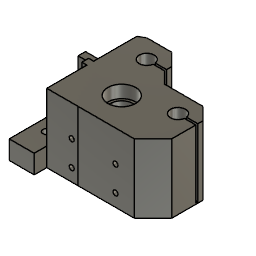
rollos monut left (Autodesk Fusion 360 design; units mm, degrees)
Autodesk Fusion 360 part; units mm, degrees
sketch "Szkic1" plane through (0, 0, 0) normal (0, 0, 1) x (1, 0, 0)
  line L0 (50, 25) -> (25, 25)
  line L1 (-35, -5) -> (-55, -5)
  line L2 (-15, 34.2) -> (0, 34.2)
  line L3 (0, 0) -> (0, -25)
  line L4 (-15.5, -15.5) -> (15.5, 15.5) construction
  line L5 (25, -25) -> (25, 25)
  line L6 (15.5, -15.5) -> (-15.5, 15.5) construction
  line L7 (-30, 25) -> (-30, 50)
  line L8 (-55, -25) -> (-55, -5)
  line L9 (-55, -5) -> (-55, 35)
  circle A0 centre (35, 10) radius 6
  line L10 (50, -5) -> (22, -5)
  line L11 (-25, 25) -> (-30, 25)
  line L12 (35, 9.2) -> (50, 9.2)
  line L13 (-25, -25) -> (-35, -25)
  line L14 (-35, -25) -> (-55, -25)
  line L15 (-40, -12.5) -> (-40, -17.5)
  line L16 (-40, -17.5) -> (-35, -17.5)
  line L17 (-40, -12.5) -> (-35, -12.5)
  line L18 (-15, 35.8) -> (0, 35.8)
  line L19 (-22, 22) -> (22, -22) construction
  line L20 (-25, -25) -> (25, -25)
  line L21 (-30, 50) -> (0, 50)
  line L22 (25, 25) -> (-25, 25)
  line L23 (22, 22) -> (-22, -22) construction
  circle A1 centre (-15, 35) radius 6
  line L24 (-35, -5) -> (-35, -25)
  line L25 (0, 50) -> (0, 25)
  circle A2 centre (-45, -15) radius 3
  line L26 (50, -5) -> (50, 25)
  line L27 (35, 10.8) -> (50, 10.8)
  line L28 (-55, 35) -> (-30, 35)
  line L29 (-25, 25) -> (-25, -25)
  circle A3 centre (0, 0) radius 11.5
  line L30 (-55, -25) -> (-55, -60)
  line L31 (-55, -60) -> (-35, -60)
  line L32 (-35, -60) -> (-35, -25)
  circle A4 centre (-45, -45) radius 3
  line L33 (50, -5) -> (25, -25)
  line L34 (-30, 50) -> (-55, 35)
  line L35 (-25, -25) -> (-25, -60)
  line L36 (-25, -60) -> (-35, -60)
  dimension "d2" = 12
  dimension "d3" = 12
  dimension "d5" = 25
  dimension "d10" = 6
  dimension "d11" = 23
  dimension "d12" = 6
  constraint coincident L3.start L23
  constraint coincident L3.start L19
  constraint perpendicular L11 L29
  constraint perpendicular L7 L11
  constraint perpendicular L7 L21
  constraint midpoint L25.end L22
  constraint perpendicular L22 L25
  constraint perpendicular L3 L20
  constraint vertical L24
  constraint coincident L3.start L6
  constraint coincident L3.start L4
  constraint coincident L6.start L19
  constraint coincident L17.end L24
  constraint perpendicular L17 L24
  constraint coincident L16.end L24
  constraint perpendicular L16 L24
  constraint perpendicular L1 L24
  constraint perpendicular L1 L9
  constraint coincident L28.end L7
  constraint perpendicular L7 L28
  constraint perpendicular L14 L24
  constraint perpendicular L8 L14
  constraint coincident L3.start A3.centre
  constraint perpendicular L14 L30
  constraint perpendicular L30 L31
  constraint perpendicular L14 L32
  constraint perpendicular L13 L35
  constraint perpendicular L32 L36
  measures "d2" diameter of A0
  measures "d3" diameter of A1
  measures "d5" distance of L3.start L3.end
  measures "d10" diameter of A2
  measures "d11" diameter of A3
  measures "d12" diameter of A4
extrude "Wyciągnięcie proste1" add sketch "Szkic1" along normal blind 10 contours L0 L5 A0 L10 L12 L26 L27 | L5 L20 L22 L29 | L5 L10 L33 | L2 L7 L11 L18 L21 L22 A1 L25 | L1 L7 L9 L11 L13 L24 L28 L29 | L13 L32 L35 L36 | L7 L28 L34 makes body 1
extrude "Wyciągnięcie proste2" add sketch "Szkic1" along normal blind 10 contours L15 L16 L17 L24 bodies 1
extrude "Wyciągnięcie proste3" add sketch "Szkic1" against normal blind 10 contours L15 L16 L17 L24 bodies 1
extrude "Wyciągnięcie proste4" add sketch "Szkic1" against normal blind 10 separate body contours L14 L30 L31 L32 makes body 2
extrude "Wyciągnięcie proste5" add sketch "Szkic1" against normal blind 10 contours L1 L8 L14 L15 L16 L17 L24 bodies 1 2
extrude "Wyciągnięcie proste6" add sketch "Szkic1" against normal blind 15 contours L0 L5 A0 L10 L12 L26 L27 | L5 L20 L22 L29 | L5 L10 L33 | L2 L7 L11 L18 L21 L22 A1 L25 | L1 L7 L9 L11 L13 L24 L28 L29 | L13 L32 L35 L36 | L7 L28 L34 bodies 1
sketch "Szkic2" plane through (0, 0, -15) normal (0, 0, -1) x (1, 0, 0)
  circle A0 centre (0, 0) radius 11.5
  line L0 (25, 25) -> (-25, 25)
  line L1 (-25, 25) -> (-25, 60)
  line L2 (-25, 60) -> (-35, 60)
  line L3 (-35, 60) -> (-35, 5)
  line L4 (-35, 5) -> (-55, 5)
  line L5 (-55, 5) -> (-55, -35)
  line L6 (-55, -35) -> (-30, -50)
  line L7 (-30, -50) -> (0, -50)
  line L8 (0, -50) -> (0, -35.8)
  line L9 (0, -35.8) -> (-9.0536, -35.8)
  arc A1 (-9.0536, -34.2) -> (-9.0536, -35.8) centre (-15, -35) ccw
  line L10 (-9.0536, -34.2) -> (0, -34.2)
  line L11 (0, -34.2) -> (0, -25)
  line L12 (0, -25) -> (25, -25)
  line L13 (25, -25) -> (50, -25)
  line L14 (50, -25) -> (50, -10.8)
  line L15 (50, -10.8) -> (40.9464, -10.8)
  arc A2 (40.9464, -9.2) -> (40.9464, -10.8) centre (35, -10) ccw
  line L16 (40.9464, -9.2) -> (50, -9.2)
  line L17 (50, -9.2) -> (50, 5)
  line L18 (50, 5) -> (25, 25)
  circle A3 centre (0, 0) radius 9
  dimension "d25" = 18
  constraint coincident A0.centre A3.centre
  measures "d25" diameter of A3
extrude "Wyciągnięcie proste7" add sketch "Szkic2" against normal blind 15 contours A0 bodies 1
chamfer "Fazowanie1" distance 9.2 angle 45 1 edges at (0, 25, -2.5) on bodies 1
chamfer "Fazowanie2" distance 10 angle 45 1 edges at (50, 25, -2.5) on bodies 1
chamfer "Fazowanie3" distance 10 angle 45 1 edges at (0, 50, -2.5) on bodies 1
chamfer "Fazowanie4" distance 15 angle 45 1 edges at (-25, -25, -2.5) on bodies 1
sketch "Szkic3" plane through (0, 0, 10) normal (0, 0, 1) x (-1, 0, 0)
  line L0 (0, -40) -> (10, -50)
  line L1 (10, -50) -> (30, -50)
  line L2 (30, -50) -> (55, -35)
  line L3 (55, -35) -> (55, 5)
  line L4 (55, 5) -> (35, 5)
  line L5 (35, 5) -> (35, 12.5)
  line L6 (35, 12.5) -> (40, 12.5)
  line L7 (40, 12.5) -> (40, 17.5)
  line L8 (40, 17.5) -> (35, 17.5)
  line L9 (35, 17.5) -> (35, 60)
  line L10 (35, 60) -> (25, 60)
  line L11 (25, 60) -> (25, 40)
  line L12 (25, 40) -> (10, 25)
  line L13 (10, 25) -> (-25, 25)
  line L14 (-25, 25) -> (-50, 5)
  line L15 (-50, 5) -> (-50, -9.2)
  line L16 (-50, -9.2) -> (-40.9464, -9.2)
  arc A0 (-40.9464, -10.8) -> (-40.9464, -9.2) centre (-35, -10) ccw
  line L17 (-40.9464, -10.8) -> (-50, -10.8)
  line L18 (-50, -10.8) -> (-50, -15)
  line L19 (-50, -15) -> (-40, -25)
  line L20 (-40, -25) -> (-25, -25)
  line L21 (-25, -25) -> (-9.2, -25)
  line L22 (-9.2, -25) -> (0, -34.2)
  line L23 (0, -34.2) -> (9.0536, -34.2)
  arc A1 (9.0536, -35.8) -> (9.0536, -34.2) centre (15, -35) ccw
  line L24 (9.0536, -35.8) -> (0, -35.8)
  line L25 (0, -35.8) -> (0, -40)
  circle A2 centre (0, 0) radius 11.5
  line L26 (55, 5) -> (35, 5)
  line L27 (35, 5) -> (35, -5)
  line L28 (35, -5) -> (55, -5)
  line L29 (55, -5) -> (55, 5)
  constraint perpendicular L26 L27
  constraint parallel L26 L28
  constraint parallel L27 L29
  constraint coincident L4.end L5.start
  constraint perpendicular L5 L26
  constraint coincident L3.end L4.start
extrude "Wyciągnięcie proste8" add sketch "Szkic3" along normal blind 25 contours L3 L4 L26 L27 L28 L29 bodies 1
sketch "Szkic4" plane through (0, 5, 0) normal (0, 1, 0) x (-1, 0, 0)
  line L0 (35, 10) -> (55, 10)
  line L1 (55, 10) -> (55, 35)
  line L2 (55, 35) -> (35, 35)
  line L3 (35, 35) -> (35, 10)
  circle A0 centre (45, 25) radius 3
  dimension "d34" = 6
  measures "d34" diameter of A0
extrude "Wyciągnięcie proste9" cut sketch "Szkic4" against normal blind 23 contours A0 bodies 1
chamfer "Fazowanie5" distance 5 angle 45 1 edges at (-45, 5, 10) on bodies 1
sketch "Szkic5" plane through (0, 0, -15) normal (0, 0, -1) x (1, 0, 0)
  circle A0 centre (0, 0) radius 9
  line L0 (-10, -50) -> (0, -40)
  line L1 (0, -40) -> (0, -35.8)
  line L2 (0, -35.8) -> (-9.0536, -35.8)
  arc A1 (-9.0536, -34.2) -> (-9.0536, -35.8) centre (-15, -35) ccw
  line L3 (-9.0536, -34.2) -> (0, -34.2)
  line L4 (0, -34.2) -> (9.2, -25)
  line L5 (9.2, -25) -> (25, -25)
  line L6 (25, -25) -> (40, -25)
  line L7 (40, -25) -> (50, -15)
  line L8 (50, -15) -> (50, -10.8)
  line L9 (50, -10.8) -> (40.9464, -10.8)
  arc A2 (40.9464, -9.2) -> (40.9464, -10.8) centre (35, -10) ccw
  line L10 (40.9464, -9.2) -> (50, -9.2)
  line L11 (50, -9.2) -> (50, 5)
  line L12 (50, 5) -> (25, 25)
  line L13 (25, 25) -> (-10, 25)
  line L14 (-10, 25) -> (-25, 40)
  line L15 (-25, 40) -> (-25, 60)
  line L16 (-25, 60) -> (-35, 60)
  line L17 (-35, 60) -> (-35, 5)
  line L18 (-35, 5) -> (-55, 5)
  line L19 (-55, 5) -> (-55, -35)
  line L20 (-55, -35) -> (-30, -50)
  line L21 (-30, -50) -> (-10, -50)
  line L22 (-9.0536, -34.2) -> (0, -34.2)
  line L23 (0, -34.2) -> (0, -35.8)
  line L24 (0, -35.8) -> (-9.0536, -35.8)
  line L25 (-9.0536, -35.8) -> (-9.0536, -34.2)
  line L26 (40.9464, -9.2) -> (50, -9.2)
  line L27 (50, -9.2) -> (50, -10.8)
  line L28 (50, -10.8) -> (40.9464, -10.8)
  line L29 (40.9464, -10.8) -> (40.9464, -9.2)
  constraint perpendicular L22 L23
  constraint parallel L22 L24
  constraint parallel L23 L25
  constraint coincident L3.end L4.start
  constraint parallel L3 L22
  constraint coincident A1.start L3.start
  constraint perpendicular L26 L27
  constraint parallel L26 L28
  constraint parallel L27 L29
  constraint perpendicular L11 L26
  constraint coincident A2.start L10.start
extrude "Wyciągnięcie proste10" add sketch "Szkic5" against normal blind 1 contours L2 L3 L22 L23 L24 L25 | L9 L10 L26 L27 L28 L29 bodies 1
sketch "Szkic6" plane through (0, -5, 0) normal (0, -1, 0) x (1, 0, 0)
  circle A0 centre (-45, 25) radius 3
  line L0 (-55, 0) -> (-35, 0)
  line L1 (-35, 0) -> (-35, 10)
  line L2 (-35, 10) -> (-35, 35)
  line L3 (-35, 35) -> (-55, 35)
  line L4 (-55, 35) -> (-55, 0)
  line L5 (-46.5, 28) -> (-43.5, 28)
  line L6 (-46.5, 28) -> (-46.5, 27)
  line L7 (-43.5, 28) -> (-43.5, 26.9)
  constraint horizontal L5
  constraint perpendicular L5 L6
  constraint perpendicular L5 L7
extrude "Wyciągnięcie proste11" cut sketch "Szkic6" against normal blind 14.2 contours A0 L5 L7 | A0 L5 L6 bodies 1
sketch "Szkic7" plane through (0, 0, -10) normal (0, 0, -1) x (1, 0, 0)
  circle A0 centre (-45, 15) radius 3
  circle A1 centre (-45, 45) radius 3
  line L0 (-35, 5) -> (-35, 60)
  line L1 (-35, 60) -> (-55, 60)
  line L2 (-55, 60) -> (-55, 5)
  line L3 (-55, 5) -> (-35, 5)
  circle A2 centre (-45, 15) radius 5.5
  circle A3 centre (-45, 45) radius 5.5
  dimension "d42" = 11
  dimension "d43" = 11
  constraint concentric A0 A2
  constraint concentric A1 A3
  measures "d42" diameter of A2
  measures "d43" diameter of A3
extrude "Wyciągnięcie proste12" add sketch "Szkic7" along normal blind 5 contours L0 L1 L2 L3 bodies 1
extrude "Wyciągnięcie proste13" add sketch "Szkic7" along normal blind 0.2 contours A0 | A1 | A2 | A3 bodies 1
sketch "Szkic8" plane through (0, 0, 0) normal (0, 0, 1) x (-1, 0, 0)
  circle A0 centre (0, 0) radius 9
  circle A1 centre (0, 0) radius 11.5
  circle A2 centre (0, 0) radius 11.5
  circle A3 centre (0, 0) radius 11.1
  dimension "d48" = 23
  dimension "d49" = 22.2
  constraint coincident A0.centre A1.centre
  measures "d48" diameter of A2
  measures "d49" diameter of A3
extrude "Wyciągnięcie proste14" add sketch "Szkic8" along normal blind 10 contours A1 A2 bodies 1
extrude "Wyciągnięcie proste15" cut 1 faces at (-45.2225, -5, 10.6917) along direction (0, 1, 0) blind 25 on bodies 1 bodies 1
extrude "Wyciągnięcie proste16" cut 1 faces at (-40, -14.1667, 6.6667) along direction (1, 0, 0) blind 5 on bodies 1 bodies 1
sketch "Szkic9" plane through (0, 0, 0) normal (0, 0, 1) x (-1, 0, 0)
  circle A0 centre (45, 15) radius 3
  circle A1 centre (45, 45) radius 3
  line L0 (35, 60) -> (35, -20)
  line L1 (35, -20) -> (55, -20)
  line L2 (55, -20) -> (55, 60)
  line L3 (55, 60) -> (35, 60)
  circle A2 centre (45, -10) radius 3
  line L4 (35, -12.5) -> (35, -7.1435)
  line L5 (35, -7.1435) -> (39, -7.1435)
  line L6 (39, -7.1435) -> (39, -12.5)
  line L7 (39, -12.5) -> (35, -12.5)
  dimension "d56" = 6
  dimension "d57" = 4
  constraint perpendicular L4 L5
  constraint parallel L4 L6
  constraint parallel L5 L7
  constraint coincident L0 L4.end
  constraint coincident L0 L4.start
  measures "d56" diameter of A2
  measures "d57" distance of L4.start L6.end
extrude "Wyciągnięcie proste17" add sketch "Szkic9" along normal blind 10 contours L0 L4 L5 L6 L7 bodies 1
extrude "Wyciągnięcie proste18" cut sketch "Szkic9" against normal blind 50 contours A2 bodies 1
sketch "Szkic10" plane through (0, 0, 10) normal (0, 0, 1) x (-1, 0, 0)
  line L0 (35, -20) -> (35, -12.5)
  line L1 (35, -12.5) -> (39, -12.5)
  line L2 (39, -12.5) -> (39, -7.1435)
  line L3 (39, -7.1435) -> (35, -7.1435)
  line L4 (35, -7.1435) -> (35, 60)
  line L5 (35, 60) -> (25, 60)
  line L6 (25, 60) -> (25, 40)
  line L7 (25, 40) -> (10, 25)
  line L8 (10, 25) -> (-25, 25)
  line L9 (-25, 25) -> (-50, 5)
  line L10 (-50, 5) -> (-50, -9.2)
  line L11 (-50, -9.2) -> (-40.9464, -9.2)
  arc A0 (-40.9464, -10.8) -> (-40.9464, -9.2) centre (-35, -10) ccw
  line L12 (-40.9464, -10.8) -> (-50, -10.8)
  line L13 (-50, -10.8) -> (-50, -15)
  line L14 (-50, -15) -> (-40, -25)
  line L15 (-40, -25) -> (-25, -25)
  line L16 (-25, -25) -> (-9.2, -25)
  line L17 (-9.2, -25) -> (0, -34.2)
  line L18 (0, -34.2) -> (9.0536, -34.2)
  arc A1 (9.0536, -35.8) -> (9.0536, -34.2) centre (15, -35) ccw
  line L19 (9.0536, -35.8) -> (0, -35.8)
  line L20 (0, -35.8) -> (0, -40)
  line L21 (0, -40) -> (10, -50)
  line L22 (10, -50) -> (30, -50)
  line L23 (30, -50) -> (55, -35)
  line L24 (55, -35) -> (55, -20)
  line L25 (55, -20) -> (35, -20)
  circle A2 centre (0, 0) radius 11.1
  line L26 (55, -20) -> (35, -20)
  line L27 (35, -20) -> (35, -26)
  line L28 (35, -26) -> (55, -26)
  line L29 (55, -26) -> (55, -20)
  dimension "d62" = 6
  constraint perpendicular L26 L27
  constraint parallel L26 L28
  constraint parallel L27 L29
  constraint coincident L0.start L25.end
  constraint parallel L25 L26
  constraint coincident L24.end L25.start
  measures "d62" distance of L24.end L28.end
extrude "Wyciągnięcie proste19" add sketch "Szkic10" along normal blind 20 contours L24 L25 L26 L27 L28 L29 bodies 1
sketch "Szkic11" plane through (0, 26, 0) normal (0, 1, 0) x (-1, 0, 0)
  line L0 (35, 10) -> (55, 10)
  line L1 (55, 10) -> (55, 30)
  line L2 (55, 30) -> (35, 30)
  line L3 (35, 30) -> (35, 10)
  circle A0 centre (45, 20) radius 3
  dimension "d65" = 6
  measures "d65" diameter of A0
extrude "Wyciągnięcie proste20" cut sketch "Szkic11" against normal blind 22 contours A0 bodies 1
chamfer "Fazowanie6" distance 20 angle 45 1 edges at (-35, 23, 10) on bodies 1
chamfer "Fazowanie7" distance 3 angle 45 1 edges at (-35, 26, 10) on bodies 1
extrude "Wyciągnięcie proste21" cut 2 faces at (-43.6198, -11.9935, -10.2) (-45.6698, -46.1601, -10.2) along direction (0, 0, 1) blind 0.2 on bodies 1 bodies 1
sketch "Szkic12" plane through (0, 0, -15) normal (0, 0, -1) x (1, 0, 0)
  circle A0 centre (-45, -10) radius 3
  circle A1 centre (-45, 45) radius 5.5
  circle A2 centre (-45, 15) radius 5.5
  line L0 (0, -34.2) -> (9.2, -25)
  line L1 (9.2, -25) -> (25, -25)
  line L2 (25, -25) -> (40, -25)
  line L3 (40, -25) -> (50, -15)
  line L4 (50, -15) -> (50, 5)
  line L5 (50, 5) -> (25, 25)
  line L6 (25, 25) -> (-10, 25)
  line L7 (-10, 25) -> (-25, 40)
  line L8 (-25, 40) -> (-25, 60)
  line L9 (-25, 60) -> (-55, 60)
  line L10 (-55, 60) -> (-55, -35)
  line L11 (-55, -35) -> (-30, -50)
  line L12 (-30, -50) -> (-10, -50)
  line L13 (-10, -50) -> (0, -40)
  line L14 (0, -40) -> (0, -34.2)
  line L15 (-9.0536, -34.2) -> (-9.0536, -35.8)
  arc A3 (-9.0536, -34.2) -> (-9.0536, -35.8) centre (-15, -35) ccw
  circle A4 centre (0, 0) radius 9
  line L16 (40.9464, -9.2) -> (40.9464, -10.8)
  arc A5 (40.9464, -9.2) -> (40.9464, -10.8) centre (35, -10) ccw
  circle A6 centre (-45, -10) radius 5.5
  dimension "d72" = 11
  constraint concentric A0 A6
  measures "d72" diameter of A6
extrude "Wyciągnięcie proste22" cut sketch "Szkic12" against normal blind 5 contours A6 bodies 1
extrude "Wyciągnięcie proste23" cut 3 faces at (-40.3538, 10.2732, -10) (-40.365, -14.5777, -10) (-40.365, -44.5777, -10) along direction (0, 0, 1) blind 4 on bodies 1 bodies 1
sketch "Szkic13" plane through (0, 0, -6) normal (0, 0, -1) x (1, 0, 0)
  circle A0 centre (-45, -10) radius 3
  circle A1 centre (-45, -10) radius 5.5
  circle A2 centre (-45, -10) radius 5.5
  circle A3 centre (-45, 15) radius 5.5
  circle A4 centre (-45, 45) radius 5.5
  dimension "d77" = 11
  dimension "d78" = 11
  constraint concentric A0 A2
  measures "d77" diameter of A3
  measures "d78" diameter of A4
extrude "Wyciągnięcie proste24" add sketch "Szkic13" along normal blind 0.2 contours A0 | A1 A2 | A3 | A4 bodies 1
delete_face "Usuń powierzchnię1" 1 faces at (-29.336, 28, 11) on bodies 1
sketch "Szkic14" plane through (0, 26, 0) normal (0, 1, 0) x (-1, 0, 0)
  circle A0 centre (45, 20) radius 3
  line L0 (55, 10) -> (55, 30)
  line L1 (55, 30) -> (35, 30)
  line L2 (35, 30) -> (15, 10)
  line L3 (15, 10) -> (55, 10)
  line L4 (15, 10) -> (35, 10)
  line L5 (35, 10) -> (35, 30)
  line L6 (35, 30) -> (15, 30)
  line L7 (15, 30) -> (15, 10)
  constraint perpendicular L4 L5
  constraint parallel L4 L6
  constraint parallel L5 L7
  constraint midpoint L3 L4.end
  constraint parallel L3 L4
  constraint coincident L2.end L3.start
extrude "Wyciągnięcie proste25" cut sketch "Szkic14" against normal blind 22 contours L2 L3 L4 L5 bodies 1
sketch "Szkic15" plane through (0, 0, 10) normal (0, 0, 1) x (-1, 0, 0)
  circle A0 centre (0, 0) radius 11.1
  line L0 (35, -12.5) -> (39, -12.5)
  line L1 (39, -12.5) -> (39, -7.1435)
  line L2 (39, -7.1435) -> (35, -7.1435)
  line L3 (35, -7.1435) -> (35, 60)
  line L4 (35, 60) -> (25, 60)
  line L5 (25, 60) -> (25, 40)
  line L6 (25, 40) -> (10, 25)
  line L7 (10, 25) -> (-25, 25)
  line L8 (-25, 25) -> (-50, 5)
  line L9 (-50, 5) -> (-50, -9.2)
  line L10 (-50, -9.2) -> (-40.9464, -9.2)
  arc A1 (-40.9464, -10.8) -> (-40.9464, -9.2) centre (-35, -10) ccw
  line L11 (-40.9464, -10.8) -> (-50, -10.8)
  line L12 (-50, -10.8) -> (-50, -15)
  line L13 (-50, -15) -> (-40, -25)
  line L14 (-40, -25) -> (-25, -25)
  line L15 (-25, -25) -> (-9.2, -25)
  line L16 (-9.2, -25) -> (0, -34.2)
  line L17 (0, -34.2) -> (9.0536, -34.2)
  arc A2 (9.0536, -35.8) -> (9.0536, -34.2) centre (15, -35) ccw
  line L18 (9.0536, -35.8) -> (0, -35.8)
  line L19 (0, -35.8) -> (0, -40)
  line L20 (0, -40) -> (10, -50)
  line L21 (10, -50) -> (30, -50)
  line L22 (30, -50) -> (55, -35)
  line L23 (55, -35) -> (55, -26)
  line L24 (55, -26) -> (35, -26)
  line L25 (35, -26) -> (35, -20)
  line L26 (35, -20) -> (35, -12.5)
  line L27 (35, -26) -> (35, -47)
  line L28 (40, -44) -> (40, -26)
  line L29 (40, -44) -> (35, -47)
  line L30 (40, -44) -> (35, -44)
  constraint coincident L24.end L25.start
  constraint coincident L22 L27.end
  constraint perpendicular L24 L27
  constraint coincident L22 L28.start
  constraint coincident L24 L28.end
  constraint perpendicular L24 L28
  constraint coincident L27 L30.end
  constraint perpendicular L27 L30
extrude "Wyciągnięcie proste26" add sketch "Szkic15" along normal blind 20 contours L24 L27 L28 L30 bodies 1
chamfer "Fazowanie8" distance 18 angle 45 1 edges at (-37.5, 44, 30) on bodies 1
chamfer "Fazowanie9" distance 2 angle 45 1 edges at (-37.5, 44, 10) on bodies 1
extrude "Wyciągnięcie proste27" cut 1 faces at (-40, 32, 17.3333) along direction (1, 0, 0) blind 1 on bodies 1 bodies 1
extrude "Wyciągnięcie proste28" cut 1 faces at (-39.6667, 44, 10.6667) along direction (0, 1, 0) blind 2.5 on bodies 1 bodies 1
extrude "Wyciągnięcie proste29" cut 1 faces at (-38.3333, -60, -10) along direction (0, 1, 0) blind 25 on bodies 1 bodies 1
extrude "Wyciągnięcie proste30" cut 1 faces at (-25, -38.3333, -6.6667) along direction (1, 0, 0) blind 10 on bodies 1 bodies 1
sketch "Szkic16" plane through (0, 0, -15) normal (0, 0, -1) x (1, 0, 0)
  line L0 (40.9464, -9.2) -> (40.9464, -10.8)
  arc A0 (40.9464, -9.2) -> (40.9464, -10.8) centre (35, -10) ccw
  circle A1 centre (0, 0) radius 9
  line L1 (-9.0536, -34.2) -> (-9.0536, -35.8)
  arc A2 (-9.0536, -34.2) -> (-9.0536, -35.8) centre (-15, -35) ccw
  circle A3 centre (-45, 15) radius 5.5
  circle A4 centre (-45, -10) radius 5.5
  line L2 (-20, 35) -> (-55, 35)
  line L3 (-55, 35) -> (-55, -35)
  line L4 (-55, -35) -> (-30, -50)
  line L5 (-30, -50) -> (-10, -50)
  line L6 (-10, -50) -> (0, -40)
  line L7 (0, -40) -> (0, -34.2)
  line L8 (0, -34.2) -> (9.2, -25)
  line L9 (9.2, -25) -> (25, -25)
  line L10 (25, -25) -> (40, -25)
  line L11 (40, -25) -> (50, -15)
  line L12 (50, -15) -> (50, 5)
  line L13 (50, 5) -> (25, 25)
  line L14 (25, 25) -> (-10, 25)
  line L15 (-10, 25) -> (-20, 35)
  line L16 (-1.2574, -54.1716) -> (43.5651, -24.2899)
  arc A5 (41.4731, -18.2674) -> (40.1418, -19.1549) centre (35, -10) ccw
  arc A6 (-8.5269, -43.2674) -> (-9.8582, -44.1549) centre (-15, -35) ccw
  line L17 (-10, -60) -> (-2.5887, -55.0591)
  line L18 (-25, -60) -> (-10, -60)
  line L19 (-35, -50) -> (-25, -60)
  line L20 (-35, -25) -> (-35, -50)
  line L21 (-25, -15) -> (-35, -25)
  line L22 (-25, -12) -> (-25, -15)
  line L23 (-18.3916, -7.3031) -> (-24.9814, -11.9814)
  line L24 (-5.2386, -11.8978) -> (-18.3916, -7.3031)
  arc A7 (-5.2386, -11.8978) -> (5, 12) centre (0, 0) ccw
  line L25 (39, 12) -> (5, 12)
  line L26 (175, 12) -> (39, 12)
  line L27 (44.8964, -23.4024) -> (65, -10)
  line L28 (65, -10) -> (175, -10)
  line L29 (175, -10) -> (175, 12)
  line L30 (5, 12) -> (-35, 12)
  line L31 (-35, 12) -> (-35, -25)
  line L32 (35, -10) -> (35, 35)
  line L33 (-55, 35) -> (-35, 35)
  line L34 (-35, 35) -> (-35, 25)
  line L35 (-35, 25) -> (-10, 25)
  constraint parallel L25 L30
  constraint coincident A0.centre A5.centre
  constraint perpendicular L25 L32
  constraint coincident L2.end L3.start
  constraint coincident L2 L33.end
  constraint perpendicular L33 L34
  constraint coincident L14.end L15.start
extrude "Wyciągnięcie proste31" cut sketch "Szkic16" against normal blind 105 contours L2 L15 L34 L35 bodies 1
sketch "Szkic17" plane through (0, -25, 0) normal (0, -1, 0) x (1, 0, 0)
  line L0 (-10, 10) -> (-35, 10)
  line L1 (-35, 10) -> (-35, 0)
  line L2 (-35, 0) -> (-35, -15)
  line L3 (-35, -15) -> (-10, -15)
  line L4 (-10, -15) -> (-10, 10)
  circle A0 centre (-15, -5) radius 2
  circle A1 centre (20, -5) radius 2
  circle A2 centre (-15, 15) radius 2
  circle A3 centre (20, 15) radius 2
  dimension "d97" = 4
  dimension "d98" = 4
  dimension "d99" = 4
  dimension "d100" = 4
  measures "d97" diameter of A0
  measures "d98" diameter of A1
  measures "d99" diameter of A2
  measures "d100" diameter of A3
extrude "Wyciągnięcie proste32" add 1 faces at (-26.992, -4.0036, 10) along direction (0, 0, 1) blind 15 on bodies 1 bodies 1
extrude "Wyciągnięcie proste33" cut sketch "Szkic17" against normal blind 10 contours A0 | A1 | A2 | A3 bodies 1
delete_face "Usuń powierzchnię2" 1 faces at (41.6667, -11.6667, -1.6667) on bodies 1
chamfer "Fazowanie10" distance 15 distance2 15 1 edges at (50, -25, 5) measured on face at (50, -13.6, -1.3333) on bodies 1
extrude "Wyciągnięcie proste34" add 1 faces at (-10.3252, 0.9986, 0) along direction (0, 0, 1) blind 15 on bodies 1 bodies 1
extrude "Wyciągnięcie proste35" add 1 faces at (25.7605, -8.3882, 25) along direction (0, 0, 1) blind 15 on bodies 1 bodies 1
extrude "Wyciągnięcie proste36" add 1 faces at (-10.3252, 0.9986, 15) along direction (0, 0, 1) blind 15 on bodies 1 bodies 1
extrude "Wyciągnięcie proste37" cut 1 faces at (-36.1111, 46, 20) along direction (0, 1, 0) blind 5 on bodies 1 bodies 1
